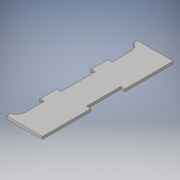
# Autodesk Inventor part: Deslizador
Saved by Autodesk Inventor 2016 (Build 200138000, 138)
## iProperties
Created: 2015-08-31
Part Number: Deslizador
Material: Generic
Document SubType Name: Modeling
Designer: amatiasq
Density: 1 g/cm^3
Appearance: Default
Author: amatiasq
Autodesk Inventor part; units mm, degrees
ref_plane "YZ Plane" through (0, 0, 0) normal (1, 0, 0) x (0, 1, 0)
ref_plane "XZ Plane" through (0, 0, 0) normal (0, 1, 0) x (-1, 0, 0)
ref_plane "XY Plane" through (0, 0, 0) normal (0, 0, 1) x (1, 0, 0)
sketch "Sketch2" plane through (0, 0, 0) normal (0, 1, 0) x (-1, 0, 0)
  line L0 (0, 0) -> (-30, 0)
  line L1 (-30, 0) -> (-30, -154)
  line L2 (-30, -154) -> (0, -154)
  line L3 (0, -154) -> (0, 0)
  line L4 (0, 0) -> (7, 0)
  line L5 (7, 0) -> (7, -5)
  arc A0 (7, -5) -> (0, -14.5394) centre (10, -14.5394) ccw
  line L6 (0, -154) -> (7, -154)
  line L7 (7, -154) -> (7, -149)
  arc A1 (0, -139.4606) -> (7, -149) centre (10, -139.4606) ccw
  line L8 (-30, 0) -> (-35, 0)
  line L9 (-35, 0) -> (-35, -57)
  line L10 (-35, -57) -> (-30, -57)
  line L11 (-30, -57) -> (-30, 0)
  line L12 (-30, -154) -> (-35, -154)
  line L13 (-35, -154) -> (-35, -97)
  line L14 (-35, -97) -> (-30, -97)
  line L15 (-30, -97) -> (-30, -154)
  line L16 (5, -37) -> (0, -37)
  line L17 (0, -57) -> (5, -57)
  line L18 (5, -57) -> (5, -37)
  line L19 (5, -97) -> (0, -97)
  line L20 (0, -117) -> (5, -117)
  line L21 (5, -117) -> (5, -97)
  dimension "d0" = 154
  dimension "d1" = 30
  dimension "d2" = 5
  dimension "d3" = 7
  dimension "d4" = 10
  dimension "d5" = 7
  dimension "d6" = 5
  dimension "d9" = 10
  dimension "d10" = 5
  dimension "d11" = 5
  dimension "d12" = 40
  dimension "d13" = 40
  dimension "d14" = 5
  dimension "d15" = 5
  dimension "d16" = 20
  dimension "d17" = 20
  constraints: 44 end point, 8 parallel, 7 horizontal, 6 point on line, 5 perpendicular, 4 point on circle, 2 centre point, 2 collinear, 2 tangent
  measures "d0" distance between parallel lines of L2 L0
  measures "d1" distance between parallel lines of L3 L1
  measures "d2" distance of L4.end L5.end
  measures "d3" distance of L4.end L0.start
  measures "d4" radius of A0
  measures "d5" distance of L2.end L6.end
  measures "d6" distance of L6.end L7.end
  measures "d9" radius of A1
  measures "d10" distance between parallel lines of L1 L9
  measures "d11" distance between parallel lines of L1 L13
  measures "d12" distance between parallel lines of L14 L10
  measures "d13" distance between parallel lines of L19 L17
  measures "d14" distance between parallel lines of L18 L3
  measures "d15" distance between parallel lines of L21 L3
  measures "d16" distance between parallel lines of L17 L16
  measures "d17" distance between parallel lines of L20 L19
extrude "cuerpo" add sketch "Sketch2" along normal blind 3
equation "\"d0\" = deslizador_largo"
equation "\"d1\" = deslizador_ancho"
equation "\"d2\" = deslizador_interruptor_largo"
equation "\"d3\" = deslizador_interruptor_ancho"
equation "\"d4\" = deslizador_interruptor_angulo"
equation "\"d5\" = d3"
equation "\"d6\" = d2"
equation "\"d9\" = d4"
equation "\"d10\" = deslizador_saliente"
equation "\"d11\" = d10"
equation "\"d12\" = movimiento_deslizador"
equation "\"d13\" = d12"
equation "\"d14\" = d10"
equation "\"d15\" = d10"
equation "\"d16\" = deslizador_saliente_largo"
equation "\"d17\" = d16"
equation "\"d18\" = deslizador_alto"
equation "\"margen\" = 0.3"
equation "\"base_alto\" = 3"
equation "\"muros_grosor\" = 3"
equation "\"rail_alto\" = 1.5"
equation "\"rail_grosor\" = 5"
equation "\"hoja_stop_posicion\" = 5"
equation "\"hoja_stop_saliente\" = 5"
equation "\"hoja_stop_largo\" = 5"
equation "\"hoja_alto\" = 3"
equation "\"hoja_stop_biselado\" = 2"
equation "\"hoja_filo_biselado\" = 0.5"
equation "\"hoja_cola_biselado\" = 1"
equation "\"deslizador_soporte_alto\" = 4"
equation "\"deslizador_tope_alto\" = 5"
equation "\"deslizador_soporte_ancho\" = 5"
equation "\"deslizador_alto\" = 3"
equation "\"tirador_agarre_largo\" = 3"
equation "\"movimiento_deslizador\" = 40"
equation "\"deslizador_largo\" = 154"
equation "\"deslizador_ancho\" = 30"
equation "\"deslizador_saliente\" = 5"
equation "\"deslizador_interruptor_angulo\" = 10"
equation "\"deslizador_interruptor_largo\" = 5"
equation "\"deslizador_interruptor_ancho\" = 7"
equation "\"deslizador_saliente_largo\" = 20"
body "Solid1"
